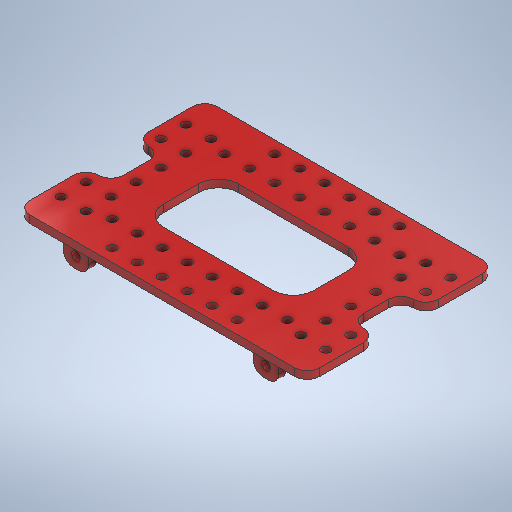
# Autodesk Inventor part: toit
Saved by Autodesk Inventor 2025 (Build 290162000, 162)
## iProperties
Created: 2024-09-16
Part Number: toit
Material: Générique
Document SubType Name: Modeling
Designer: chass
Density: 1 g/cm^3
Appearance: Par défaut
Author: chass
## iProperties of the stored document toit_Impression 3D.ipt
Created: 2024-09-16
Part Number: toit_Impression 3D
Material: Générique
Document SubType Name: Modeling
Designer: chass
Density: 1 g/cm^3
Appearance: Par défaut
Author: chass
Autodesk Inventor part; units mm, degrees
ref_plane "YZ Plane" through (0, 0, 0) normal (1, 0, 0) x (0, 1, 0)
ref_plane "XZ Plane" through (0, 0, 0) normal (0, 1, 0) x (-1, 0, 0)
ref_plane "XY Plane" through (0, 0, 0) normal (0, 0, 1) x (1, 0, 0)
sketch "Esquisse1" plane through (0, 0, 0) normal (0, 1, 0) x (-1, 0, 0)
  line L0 (58, 37.5) -> (-58, 37.5)
  line L1 (-58, 37.5) -> (-58, -37.5)
  line L2 (-58, -37.5) -> (58, -37.5)
  line L3 (58, -37.5) -> (58, 37.5)
  line L4 (58, 37.5) -> (-58, -37.5)
  line L5 (-58, 37.5) -> (58, -37.5)
  circle A0 centre (53, 25) radius 1.75
  circle A1 centre (53, 15) radius 1.75
  line L6 (67, 0) -> (-72, 0)
  circle A2 centre (43, 25) radius 1.75
  circle A3 centre (43, 15) radius 1.75
  circle A4 centre (43, 5) radius 1.75
  circle A5 centre (53, -25) radius 1.75
  circle A6 centre (53, -15) radius 1.75
  circle A7 centre (43, -25) radius 1.75
  circle A8 centre (43, -15) radius 1.75
  circle A9 centre (43, -5) radius 1.75
  line L7 (0, 59.5) -> (0, -79.5)
  circle A10 centre (-53, 25) radius 1.75
  circle A11 centre (-53, 15) radius 1.75
  circle A12 centre (-43, 25) radius 1.75
  circle A13 centre (-43, 15) radius 1.75
  circle A14 centre (-43, 5) radius 1.75
  circle A15 centre (-43, -25) radius 1.75
  circle A16 centre (-43, -15) radius 1.75
  circle A17 centre (-53, -15) radius 1.75
  circle A18 centre (-43, -5) radius 1.75
  circle A19 centre (-53, -25) radius 1.75
  circle A20 centre (5, 32.5) radius 1.75
  circle A21 centre (5, 22.5) radius 1.75
  circle A22 centre (15, 32.5) radius 1.75
  circle A23 centre (15, 22.5) radius 1.75
  circle A24 centre (25, 32.5) radius 1.75
  circle A25 centre (25, 22.5) radius 1.75
  circle A26 centre (35, 22.5) radius 1.75
  circle A27 centre (-5, 32.5) radius 1.75
  circle A28 centre (-5, 22.5) radius 1.75
  circle A29 centre (-15, 32.5) radius 1.75
  circle A30 centre (-15, 22.5) radius 1.75
  circle A31 centre (-25, 32.5) radius 1.75
  circle A32 centre (-25, 22.5) radius 1.75
  circle A33 centre (-35, 22.5) radius 1.75
  circle A34 centre (5, -32.5) radius 1.75
  circle A35 centre (5, -22.5) radius 1.75
  circle A36 centre (15, -32.5) radius 1.75
  circle A37 centre (15, -22.5) radius 1.75
  circle A38 centre (25, -32.5) radius 1.75
  circle A39 centre (25, -22.5) radius 1.75
  circle A40 centre (35, -22.5) radius 1.75
  circle A41 centre (-35, -22.5) radius 1.75
  circle A42 centre (-25, -22.5) radius 1.75
  circle A43 centre (-25, -32.5) radius 1.75
  circle A44 centre (-15, -22.5) radius 1.75
  circle A45 centre (-15, -32.5) radius 1.75
  circle A46 centre (-5, -22.5) radius 1.75
  circle A47 centre (-5, -32.5) radius 1.75
  line L8 (30, 15) -> (-30, 15)
  line L9 (-30, 15) -> (-30, -15)
  line L10 (-30, -15) -> (30, -15)
  line L11 (30, -15) -> (30, 15)
  line L12 (30, 15) -> (-30, -15)
  line L13 (-30, 15) -> (30, -15)
  line L14 (-58, 10) -> (-48, 10)
  line L15 (-48, 10) -> (-48, -10)
  line L16 (-48, -10) -> (-58, -10)
  line L17 (-58, -10) -> (-58, 10)
  line L18 (-58, 10) -> (-48, -10)
  line L19 (-48, 10) -> (-58, -10)
  line L20 (58, 10) -> (48, 10)
  line L21 (48, 10) -> (48, -10)
  line L22 (48, -10) -> (58, -10)
  line L23 (58, -10) -> (58, 10)
  line L24 (58, 10) -> (48, -10)
  line L25 (48, 10) -> (58, -10)
  point P0 (0, 0)
  point P1 (0, 0)
  point P2 (0, 0)
  point P3 (-53, 0)
  point P4 (53, 0)
  dimension "d0" = 116
  dimension "d1" = 75
  dimension "d3" = 3.5
  dimension "d4" = 3.5
  dimension "d7" = 10
  dimension "d9" = 3.5
  dimension "d10" = 3.5
  dimension "d11" = 3.5
  dimension "d12" = 10
  dimension "d13" = 10
  dimension "d15" = 5
  dimension "d16" = 5
  dimension "d17" = 5
  dimension "d19" = 3.5
  dimension "d20" = 3.5
  dimension "d21" = 3.5
  dimension "d22" = 3.5
  dimension "d23" = 3.5
  dimension "d24" = 3.5
  dimension "d26" = 3.5
  dimension "d27" = 5
  dimension "d28" = 5
  dimension "d29" = 10
  dimension "d30" = 5
  dimension "d31" = 10
  dimension "d32" = 10
  dimension "d33" = 10
  dimension "d34" = 5
  dimension "d35" = 10
  dimension "d36" = 10
  dimension "d37" = 5
  dimension "d38" = 10
  dimension "d40" = 10
  dimension "d44" = 30
  dimension "d45" = 60
  dimension "d64" = 10
  dimension "d65" = 20
  dimension "d66" = 0
  dimension "d67" = 0
  dimension "d68" = 37.5
  constraints: 52 end point, 48 centre point, 41 symmetric about line, 6 parallel, 4 midpoint, 4 perpendicular, 3 horizontal, 1 coincident, 1 vertical, 36 other
  measures "d0" distance of L2.end L1.end
  measures "d1" distance of L1.end L0.end
  measures "d3" diameter of A0
  measures "d4" diameter of A1
  measures "d7" distance of A0.centre A1.centre
  measures "d9" diameter of A2
  measures "d10" diameter of A3
  measures "d11" diameter of A4
  measures "d12" distance of A0.centre A2.centre
  measures "d13" distance of A3.centre A1.centre
  measures "d15" distance from line of L6 A4.centre
  measures "d16" distance from line of L3 A1.centre
  measures "d17" distance from line of L3 A0.centre
  measures "d19" diameter of A20
  measures "d20" diameter of A21
  measures "d21" diameter of A22
  measures "d22" diameter of A23
  measures "d23" diameter of A24
  measures "d24" diameter of A25
  measures "d26" diameter of A26
  measures "d27" distance from line of L7 A20.centre
  measures "d28" distance from line of L7 A21.centre
  measures "d29" distance of A21.centre A20.centre
  measures "d30" distance from line of L0 A20.centre
  measures "d31" distance of A20.centre A22.centre
  measures "d32" distance of A21.centre A23.centre
  measures "d33" distance of A23.centre A22.centre
  measures "d34" distance from line of L0 A22.centre
  measures "d35" distance of A22.centre A24.centre
  measures "d36" distance of A23.centre A25.centre
  measures "d37" distance from line of L0 A24.centre
  measures "d38" distance of A25.centre A24.centre
  measures "d40" distance of A26.centre A25.centre
  measures "d44" distance of L10.end L8.start
  measures "d45" distance of L9.end L10.end
  measures "d64" distance of L15.end L16.end
  measures "d65" distance of L14.end L15.end
  measures "d66" distance between parallel lines of L1 L17
  measures "d67" distance from line of L6 point (-53, 0)
  measures "d68" distance between parallel lines of L0 L6
extrude "Extrusion1" add sketch "Esquisse1" along normal blind 3 contours L4 A26 L8 L7 L0 | L3 L20 L21 L6 L11 L8 L4 A26 | L7 L8 L5 A33 L0 | L5 A33 L8 L9 L6 L15 L14 L1 | L3 L5 A40 L10 L11 L6 L21 L22 | L10 L7 L2 L4 A41 | L4 A41 L1 L16 L15 L6 L9 L10 | L5 A40 L2 L7 L10
fillet "Congé1" radius 5 4 edges at (58, 1.5, 37.5) (58, 1.5, -37.5) (-58, 1.5, -37.5) (-58, 1.5, 37.5)
fillet "Congé2" radius 8 4 edges at (-30, 1.5, -15) (-30, 1.5, 15) (30, 1.5, 15) (30, 1.5, -15)
sketch "Esquisse2" plane through (0, 0, 0) normal (0, -1, 0) x (1, 0, 0)
  line L0 (-43, 34) -> (-33, 34)
  line L1 (-33, 34) -> (-33, 31)
  line L2 (-33, 31) -> (-43, 31)
  line L3 (-43, 31) -> (-43, 34)
  line L4 (-43, 34) -> (-33, 31)
  line L5 (-43, 31) -> (-33, 34)
  line L6 (-53, 37.5) -> (53, 37.5) projected
  line L7 (-58, -32.5) -> (-58, 32.5) projected
  line L8 (-92, 0) -> (78, 0)
  line L9 (0, 51) -> (0, -66)
  line L10 (-43, -34) -> (-33, -34)
  line L11 (-33, -34) -> (-33, -31)
  line L12 (-33, -31) -> (-43, -31)
  line L13 (-43, -31) -> (-43, -34)
  line L14 (-43, -34) -> (-33, -31)
  line L15 (-43, -31) -> (-33, -34)
  line L16 (0, -51) -> (0, 66)
  line L17 (43, 34) -> (33, 34)
  line L18 (33, 34) -> (33, 31)
  line L19 (33, 31) -> (43, 31)
  line L20 (43, 31) -> (43, 34)
  line L21 (43, 34) -> (33, 31)
  line L22 (43, 31) -> (33, 34)
  line L23 (43, -34) -> (33, -34)
  line L24 (33, -34) -> (33, -31)
  line L25 (33, -31) -> (43, -31)
  line L26 (43, -31) -> (43, -34)
  line L27 (43, -34) -> (33, -31)
  line L28 (43, -31) -> (33, -34)
  point P0 (0, 0)
  point P1 (-38, 32.5)
  point P2 (-38, -32.5)
  point P3 (38, 32.5)
  point P4 (38, -32.5)
  dimension "d50" = 3
  dimension "d51" = 10
  dimension "d52" = 3.5
  dimension "d53" = 20
  constraints: 54 end point, 17 symmetric about line, 2 horizontal, 2 parallel, 2 perpendicular, 1 midpoint
  measures "d50" distance of L0.end L1.end
  measures "d51" distance of L0.start L0.end
  measures "d52" distance between parallel lines of L6 L0
  measures "d53" distance from line of L7 point (-38, 32.5)
extrude "Extrusion2" add sketch "Esquisse2" along normal blind 10
sketch "Esquisse3" plane through (-43, 0, 34) normal (0, 0, 1) x (1, 0, 0)
  circle A0 centre (5, -5.5) radius 1.75
  line L0 (-10, 3) -> (96, 3) projected
  line L1 (-10, 0) -> (96, 0) projected
  line L2 (0, 0) -> (0, -10) projected
  line L3 (43, 22) -> (43, -21)
  circle A1 centre (81, -5.5) radius 1.75
  point P0 (43, 0)
  dimension "d56" = 3.5
  dimension "d58" = 5.5
  dimension "d59" = 5
  constraints: 2 centre point, 2 end point, 1 symmetric about line, 1 vertical, 1 other
  measures "d56" diameter of A0
  measures "d58" distance from line of L1 A0.centre
  measures "d59" distance from line of L2 A0.centre
extrude "Extrusion3" cut sketch "Esquisse3" against normal blind 75.25
fillet "Congé3" radius 4 8 edges at (-43, -10, 32.5) (-33, -10, 32.5) (-33, -10, -32.5) (-43, -10, -32.5) (33, -10, -32.5) (43, -10, -32.5) (33, -10, 32.5) (43, -10, 32.5)
fillet "Congé4" radius 2 12 edges at (38, 0, 31) (43, 0, 32.5) (33, 0, 32.5) (-38, 0, 31) (-33, 0, 32.5) (-43, 0, 32.5) (-38, 0, -31) (-43, 0, -32.5) (-33, 0, -32.5) (33, 0, -32.5) (38, 0, -31) (43, 0, -32.5)
fillet "Congé5" radius 5 8 edges at (-58, 1.5, -10) (-48, 1.5, -10) (-48, 1.5, 10) (-58, 1.5, 10) (58, 1.5, 10) (48, 1.5, 10) (58, 1.5, -10) (48, 1.5, -10)
